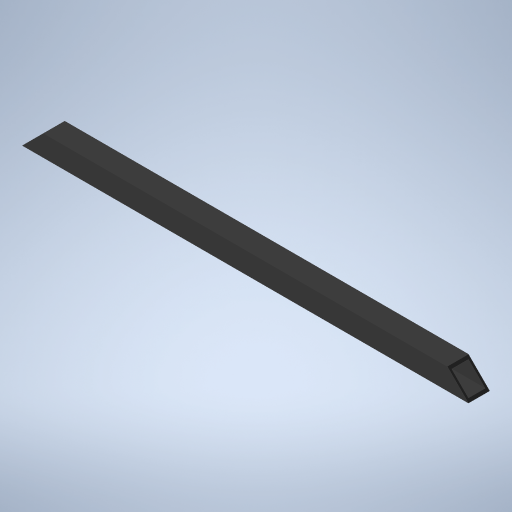
# Autodesk Inventor part: RS2_TubeFoot
Saved by Autodesk Inventor 2024.3 (Build 283343000, 343)
## iProperties
Created: 2025-04-11
Part Number: RS2_TubeFoot
Material: Generic
Document SubType Name: Modeling
Designer: ajclo
Density: 1 g/cm^3
Appearance: Default
Mass: 51.7553 g
Surface Area: 521.446 cm^2
Volume: 51.7553 cm^3
Author: ajclo
Autodesk Inventor part; units mm, degrees
ref_plane "YZ Plane" through (0, 0, 0) normal (1, 0, 0) x (0, 1, 0)
ref_plane "XZ Plane" through (0, 0, 0) normal (0, 1, 0) x (-1, 0, 0)
ref_plane "XY Plane" through (0, 0, 0) normal (0, 0, 1) x (1, 0, 0)
sketch "Sketch1" plane through (0, 0, 0) normal (1, 0, 0) x (0, 1, 0)
  line L0 (-9.5, 9.5) -> (9.5, 9.5)
  line L1 (9.5, 9.5) -> (9.5, -9.5)
  line L2 (9.5, -9.5) -> (-9.5, -9.5)
  line L3 (-9.5, -9.5) -> (-9.5, 9.5)
  line L4 (-9.5, 9.5) -> (9.5, -9.5) construction
  line L5 (9.5, 9.5) -> (-9.5, -9.5) construction
  line L6 (-7.5, 7.5) -> (7.5, 7.5)
  line L7 (7.5, 7.5) -> (7.5, -7.5)
  line L8 (7.5, -7.5) -> (-7.5, -7.5)
  line L9 (-7.5, -7.5) -> (-7.5, 7.5)
  line L10 (-7.5, 7.5) -> (7.5, -7.5) construction
  line L11 (7.5, 7.5) -> (-7.5, -7.5) construction
  point P0 (0, 0)
  dimension "d0" = 2
  dimension "d1" = 2
  dimension "d2" = 19
  dimension "d3" = 19
  constraints: 24 end point, 4 midpoint, 4 parallel, 2 horizontal, 2 perpendicular
  measures "d0" distance between parallel lines of L1 L7
  measures "d1" distance between parallel lines of L2 L8
  measures "d2" distance of L1.end L2.end
  measures "d3" distance of L0.end L1.end
extrude "Extrusion1" add sketch "Sketch1" along normal blind 400
sketch "Sketch2" plane through (0, -9.5, 9.5) normal (0, 0, 1) x (1, 0, 0)
  line L0 (0, 19) -> (0, 0) projected
  line L1 (0, 19) -> (400, 19) projected
  line L2 (400, 19) -> (400, 0) projected
  line L3 (0, 0) -> (400, 0) projected
  line L4 (0, 0) -> (19, 19)
  line L5 (400, 0) -> (381, 19)
  point P0 (0, 9.5)
  dimension "d10" = 45
  dimension "d11" = 45
  constraints: 4 end point, 2 point on line
  measures "d10" angle of L5 L3
  measures "d11" angle of L3 L4
extrude "Extrusion2" cut sketch "Sketch2" against normal through all contours L1 L4 L0 | L5 L1 L2
equation "\"d1\" = d0"
body "Solid1"
